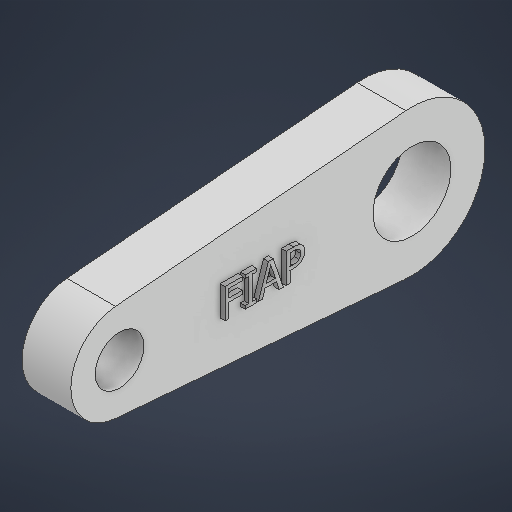
# Autodesk Inventor part: Peça1
Saved by Autodesk Inventor 2027 (Build 310192060, 192F)
## iProperties
Created: 2026-08-25
Part Number: Peça1
Material: Genérico
Document SubType Name: Modeling
Designer: guisg
Density: 1 g/cm^3
Appearance: Padrão
Author: guisg
Autodesk Inventor part; units mm, degrees
ref_plane "YZ Plane" through (0, 0, 0) normal (1, 0, 0) x (0, 1, 0)
ref_plane "XZ Plane" through (0, 0, 0) normal (0, 1, 0) x (-1, 0, 0)
ref_plane "XY Plane" through (0, 0, 0) normal (0, 0, 1) x (1, 0, 0)
sketch "Esboço1" plane through (0, 0, 0) normal (1, 0, 0) x (0, 1, 0)
  line L0 (0, 0) -> (0, 30)
  circle A0 centre (0, 0) radius 4
  circle A1 centre (0, 30) radius 2.5
  arc A2 (4.9826, 30.4167) -> (-4.9826, 30.4167) centre (0, 30) ccw
  arc A3 (-7.4739, 0.625) -> (7.4739, 0.625) centre (0, 0) ccw
  line L1 (4.9826, 30.4167) -> (7.4739, 0.625)
  line L2 (-4.9826, 30.4167) -> (-7.4739, 0.625)
  constraints: 6 end point, 5 coincident, 4 centre point, 4 point on circle, 4 tangent, 1 vertical
extrude "Extrusão1" add sketch "Esboço1" along normal mid plane 5
sketch "Esboço2" plane through (2.5, 0, 0) normal (1, 0, 0) x (0, 0, -1)
  line L0 (-19.9846, 1.6224) -> (-11.4087, 1.6224) construction
  line L1 (-11.4087, 1.6224) -> (-11.4087, -1.4256) construction
  line L2 (-11.4087, -1.4256) -> (-19.9846, -1.4256) construction
  line L3 (-19.9846, -1.4256) -> (-19.9846, 1.6224) construction
  circle A0 centre (-30, 0) radius 2.5 projected
  line L4 (-17.853, 1.2618) -> (-19.2708, 1.2618)
  line L5 (-19.2708, 1.2618) -> (-19.2708, 0.4022)
  line L6 (-19.2708, 0.4022) -> (-17.9122, 0.4022)
  line L7 (-17.9122, 0.4022) -> (-17.9122, 0.0416)
  line L8 (-17.9122, 0.0416) -> (-19.2708, 0.0416)
  line L9 (-19.2708, 0.0416) -> (-19.2708, -1.4256)
  line L10 (-19.2708, -1.4256) -> (-19.6758, -1.4256)
  line L11 (-19.6758, -1.4256) -> (-19.6758, 1.6224)
  line L12 (-19.6758, 1.6224) -> (-17.853, 1.6224)
  line L13 (-17.853, 1.6224) -> (-17.853, 1.2618)
  line L14 (-16.4278, -1.4256) -> (-17.6084, -1.4256)
  line L15 (-17.6084, -1.4256) -> (-17.6084, -1.1144)
  line L16 (-17.6084, -1.1144) -> (-17.2206, -1.1144)
  line L17 (-17.2206, -1.1144) -> (-17.2206, 1.3112)
  line L18 (-17.2206, 1.3112) -> (-17.6084, 1.3112)
  line L19 (-17.6084, 1.3112) -> (-17.6084, 1.6224)
  line L20 (-17.6084, 1.6224) -> (-16.4278, 1.6224)
  line L21 (-16.4278, 1.6224) -> (-16.4278, 1.3112)
  line L22 (-16.4278, 1.3112) -> (-16.8156, 1.3112)
  line L23 (-16.8156, 1.3112) -> (-16.8156, -1.1144)
  line L24 (-16.8156, -1.1144) -> (-16.4278, -1.1144)
  line L25 (-16.4278, -1.1144) -> (-16.4278, -1.4256)
  line L26 (-16.2549, -1.4256) -> (-15.2273, 1.6224)
  line L27 (-15.2273, 1.6224) -> (-14.7284, 1.6224)
  line L28 (-14.7284, 1.6224) -> (-13.7009, -1.4256)
  line L29 (-13.7009, -1.4256) -> (-14.1282, -1.4256)
  line L30 (-14.1282, -1.4256) -> (-14.4048, -0.5735)
  line L31 (-14.4048, -0.5735) -> (-15.5682, -0.5735)
  line L32 (-15.5682, -0.5735) -> (-15.8448, -1.4256)
  line L33 (-15.8448, -1.4256) -> (-16.2549, -1.4256)
  line L34 (-14.516, -0.2276) -> (-14.9877, 1.2074)
  line L35 (-14.9877, 1.2074) -> (-15.457, -0.2276)
  line L36 (-15.457, -0.2276) -> (-14.516, -0.2276)
  spline S0 degree 2 poles (-11.4853, 0.7035) (-11.4853, 0.5059) (-11.6261, 0.1503) (-11.752, 0.0268) knots 0 0 0 1 2 2 2
  spline S1 degree 2 poles (-11.752, 0.0268) (-11.9101, -0.1288) (-12.3374, -0.2894) (-12.6635, -0.2894) knots 0 0 0 1 2 2 2
  line L37 (-12.6635, -0.2894) -> (-13.0068, -0.2894)
  line L38 (-13.0068, -0.2894) -> (-13.0068, -1.4256)
  line L39 (-13.0068, -1.4256) -> (-13.4119, -1.4256)
  line L40 (-13.4119, -1.4256) -> (-13.4119, 1.6224)
  line L41 (-13.4119, 1.6224) -> (-12.6462, 1.6224)
  spline S2 degree 2 poles (-12.6462, 1.6224) (-12.3745, 1.6224) (-11.9941, 1.5335) (-11.8484, 1.4322) knots 0 0 0 1 2 2 2
  spline S3 degree 2 poles (-11.8484, 1.4322) (-11.6779, 1.3161) (-11.4853, 0.958) (-11.4853, 0.7035) knots 0 0 0 1 2 2 2
  spline S4 degree 2 poles (-11.9076, 0.6912) (-11.9076, 0.8493) (-12.0163, 1.0815) (-12.1275, 1.1556) knots 0 0 0 1 2 2 2
  spline S5 degree 2 poles (-12.1275, 1.1556) (-12.2238, 1.2198) (-12.4807, 1.2717) (-12.6709, 1.2717) knots 0 0 0 1 2 2 2
  line L42 (-12.6709, 1.2717) -> (-13.0068, 1.2717)
  line L43 (-13.0068, 1.2717) -> (-13.0068, 0.0564)
  line L44 (-13.0068, 0.0564) -> (-12.7302, 0.0564)
  spline S6 degree 2 poles (-12.7302, 0.0564) (-12.4831, 0.0564) (-12.1793, 0.1354) (-12.0805, 0.2392) knots 0 0 0 1 2 2 2
  spline S7 degree 2 poles (-12.0805, 0.2392) (-11.9891, 0.3306) (-11.9076, 0.5455) (-11.9076, 0.6912) knots 0 0 0 1 2 2 2
  point P0 (0, 0)
  constraints: 2 other
extrude "Extrusão2" add sketch "Esboço2" along normal blind 0.5 contours L4 L5 L6 L7 L8 L9 L10 L11 L12 L13 | L14 L15 L16 L17 L18 L19 L20 L21 L22 L23 L24 L25 | L26 L27 L28 L29 L30 L31 L32 L33 | S0 S1 L37 L38 L39 L40 L41 S2 S3
